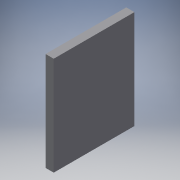
# Autodesk Inventor part: cap1
Saved by Autodesk Inventor 2018 (Build 220112000, 112)
## iProperties
Created: 2018-02-05
Part Number: cap1
Material: Generic
Document SubType Name: Modeling
Designer: Benedikt
Density: 1 g/cm^3
Appearance: Default
Author: Benedikt
Autodesk Inventor part; units mm, degrees
ref_plane "YZ Plane" through (0, 0, 0) normal (1, 0, 0) x (0, 1, 0)
ref_plane "XZ Plane" through (0, 0, 0) normal (0, 1, 0) x (-1, 0, 0)
ref_plane "XY Plane" through (0, 0, 0) normal (0, 0, 1) x (1, 0, 0)
sketch "Sketch1" plane through (0, 0, 0) normal (1, 0, 0) x (0, 1, 0)
  line L0 (0, 0) -> (7.3855, 0)
  line L1 (7.3855, 0) -> (7.3855, 9.0203)
  line L2 (7.3855, 9.0203) -> (0, 9.0203)
  line L3 (0, 9.0203) -> (0, 0)
  constraints: 8 end point, 2 parallel, 1 horizontal, 1 perpendicular
extrude "Extrusion1" add sketch "Sketch1" along normal blind 0.75
body "Solid1"
